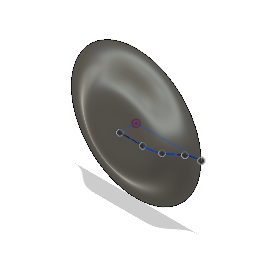
Composite01.v2 (Autodesk Fusion 360 design; units mm, degrees)
Autodesk Fusion 360 part; units mm, degrees
sketch "Sketch4" plane through (0, 0, 0) normal (0, 1, 0) x (1, 0, 0)
  spline S0 degree 5 poles (0, -25) (1.2915, -24.9531) (3.8621, -24.8698) (7.6815, -24.7768) (12.7002, -24.7168) (18.8471, -24.7416) (24.8602, -24.843) (30.7265, -24.9718) (36.427, -25.0444) (41.9351, -24.9296) (47.2169, -24.449) (52.2416, -23.4267) (56.9901, -21.7317) (61.4635, -19.3203) (65.695, -16.2916) (69.7532, -12.9013) (73.7253, -9.4764) (77.7044, -6.3493) (81.7773, -3.7917) (86.0085, -1.9298) (90.4356, -0.7321) (94.1498, -0.2225) (97.0358, -0.0405) (99.0045, 0) (100, 0) knots 0 0 0 0 0 0 0.05 0.1 0.15 0.2 0.25 0.3 0.35 0.4 0.45 0.5 0.55 0.6 0.65 0.7 0.75 0.8 0.85 0.9 0.95 1 1 1 1 1 1
  line L0 (88, 0) -> (112, 0)
  line L1 (0, 0) -> (100, 0)
  line L2 (0, 0) -> (0, -25)
  point P0 (35, -25)
  point P1 (60, -20)
  point P2 (80, -5)
  constraint midpoint S0.end L0
  constraint coincident L1.start L2.start
  constraint parallel L0 L1
  constraint perpendicular L1 L2
revolve "Revolve2" add sketch "Sketch4" angle 360 about axis through (0, 0, 1.75) along (0, 0, 1)
